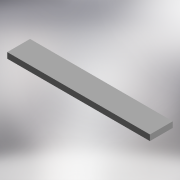
# Autodesk Inventor part: Z-encoder-mounting-plate
Saved by Autodesk Inventor 2016 (Build 200138000, 138)
## iProperties
Created: 2015-05-21
Part Number: Z-encoder-mounting-plate
Material: PC/ABS Plastic
Document SubType Name: Modeling
Designer: as
Mass: 1.5247 g
Surface Area: 24.9204 cm^2
Volume: 4.26762 cm^3
Density: 0.357273 g/cm^3
Appearance: Smooth - White
Author: as
Autodesk Inventor part; units mm, degrees
ref_plane "YZ Plane" through (0, 0, 0) normal (1, 0, 0) x (0, 1, 0)
ref_plane "XZ Plane" through (0, 0, 0) normal (0, 1, 0) x (-1, 0, 0)
ref_plane "XY Plane" through (0, 0, 0) normal (0, 0, 1) x (1, 0, 0)
sketch "Sketch1" plane through (0, 0, 0) normal (0, 0, 1) x (1, 0, 0)
  circle A0 centre (5, 8.5) radius 2.25 projected
  circle A1 centre (19, 8.5) radius 2.25 projected
  line L0 (25, 4) -> (-25, 4)
  line L1 (-25, 4) -> (-25, -4)
  line L2 (-25, -4) -> (25, -4)
  line L3 (25, -4) -> (25, 4)
  line L4 (25, 4) -> (-25, -4) construction
  line L5 (-25, 4) -> (25, -4) construction
  point P0 (0, 0)
  point P1 (-21, 0)
  point P2 (-2.5, 0)
  dimension "d39" = 50
  dimension "d40" = 8
  dimension "d41" = 4
  dimension "d42" = 18.5
  dimension "d43" = 4
  constraints: 12 end point, 2 midpoint, 2 parallel, 1 horizontal, 1 perpendicular
  measures "d39" distance of L1.end L2.end
  measures "d40" distance of L0.end L1.end
  measures "d41" distance from line of point (-21, 0) L1
  measures "d42" distance of point (-2.5, 0) point (-21, 0)
  measures "d43" distance from line of L2 point (-21, 0)
extrude "Extrusion1" add sketch "Sketch1" against normal blind 8 contours L3 L2 L1 L0
sketch "Sketch7" plane through (-25, 4, 0) normal (0, 1, 0) x (1, 0, 0)
  line L0 (50, 8) -> (30, 8)
  line L1 (30, 8) -> (30, 3)
  line L2 (30, 3) -> (50, 3)
  line L3 (50, 3) -> (50, 8)
  point P0 (25, 0)
  dimension "d44" = 20
  dimension "d45" = 5
  constraints: 8 end point, 2 parallel, 1 horizontal, 1 perpendicular
  measures "d44" distance of L2.end L1.end
  measures "d45" distance of L1.end L0.end
extrude "Extrusion3" add sketch "Sketch7" along normal blind 12
sketch "Sketch8" plane through (0, 0, -8) normal (0, 0, -1) x (-1, 0, 0)
  line L0 (25, -4) -> (25, 4) projected
  line L1 (-25, -4) -> (25, -4) projected
  point P0 (0, 0)
  point P1 (21, -1)
  point P2 (2.5, -1)
  dimension "d48" = 4
  dimension "d49" = 18.5
  dimension "d50" = 3
  dimension "d51" = 3
  measures "d48" distance from line of L0 point (21, -1)
  measures "d49" distance of point (21, -1) point (2.5, -1)
  measures "d50" distance from line of L1 point (21, -1)
  measures "d51" distance from line of L1 point (2.5, -1)
hole "Hole4" at (0, 0, -8) at (-21, -1, -8) direction (0, 0, 1) diameter 3 depth 8 tip angle 118
sketch "Sketch9" plane through (5, 4, -3) normal (0, 0, 1) x (1, 0, 0)
  point P0 (17, 3.4563)
  point P1 (3, 3.4563)
hole "Hole5" at (22, 7.4563, -3) at (8, 7.4563, -3) direction (0, 0, -1) diameter 1.567 depth 10 tip angle 120 thread size "M2x0.4" class "6H" standard "ISO Metric profile"
body "Solid1"
